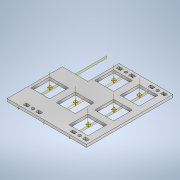
# Autodesk Inventor part: tc_base_plate
Saved by Autodesk Inventor 2020.1 (Build 241239000, 239)
## iProperties
Created: 2019-07-03
Part Number: tc_base_plate
Material: Acier inoxydable
Document SubType Name: Modeling
Designer: Thibault
Density: 8 g/cm^3
Appearance: Aluminium - Poli
Mass: 33.3223 g
Surface Area: 56.2435 cm^2
Volume: 4.16528 cm^3
tc_base_width: 59,100 mm
tc_base_back_width: 40,050 mm
tc_base_support_dist: 56,100 mm
Author: Thibault
Autodesk Inventor part; units mm, degrees
ref_plane "YZ Plane" through (0, 0, 0) normal (1, 0, 0) x (0, 1, 0)
ref_plane "XZ Plane" through (0, 0, 0) normal (0, 1, 0) x (-1, 0, 0)
ref_plane "XY Plane" through (0, 0, 0) normal (0, 0, 1) x (1, 0, 0)
sketch "screw_anchor" plane through (0, 0, 0) normal (0, 0, 1) x (1, 0, 0)
  point P0 (61.1245, 15.5217)
  dimension "d155" = 14
  dimension "d156" = 19.05
  dimension "d157" = 19.05
  dimension "d158" = 19.05
  dimension "d159" = 28.575
  dimension "d160" = 19.05
  dimension "d161" = 2
  dimension "d162" = 2
  dimension "d163" = 2
  dimension "d164" = 2
  dimension "d165" = 2
  dimension "d166" = 1
  dimension "d167" = 5
  dimension "d168" = 5
  dimension "d169" = 4
  dimension "tc_base_support_dist" = 56.1
sketch "anchor" plane through (0, 0, 0) normal (0, 0, 1) x (1, 0, 0)
  circle A0 centre (94.2814, 48.5827) radius 0.85
  line L0 (91.2814, 49.5827) -> (87.2814, 49.5827)
  line L1 (87.2814, 49.5827) -> (87.2814, 47.5827)
  line L2 (87.2814, 47.5827) -> (91.2814, 47.5827)
  line L3 (91.2814, 47.5827) -> (91.2814, 49.5827)
  line L4 (101.2814, 49.5827) -> (97.2814, 49.5827)
  line L5 (97.2814, 49.5827) -> (97.2814, 47.5827)
  line L6 (97.2814, 47.5827) -> (101.2814, 47.5827)
  line L7 (101.2814, 47.5827) -> (101.2814, 49.5827)
  line L8 (91.2814, 49.5827) -> (97.2814, 47.5827) construction
  line L9 (97.2814, 49.5827) -> (91.2814, 47.5827) construction
  line L10 (87.2814, 51.1827) -> (101.2814, 51.1827)
  point P0 (103.5798, 50.1132)
  point P1 (94.2814, 48.5827)
  dimension "tc_base_support_dist" = 56.1
  dimension "d226" = 1.7
  dimension "d230" = 4
  dimension "d231" = 2
  dimension "d237" = 4
  dimension "d245" = 1.6
  dimension "d247" = 6
  measures "d226" diameter of A0
  measures "d230" distance of L2.end L1.end
  measures "d231" distance of L1.end L0.end
  measures "d237" distance of L6.end L5.end
  measures "d245" distance between parallel lines of L0 L10
  measures "d247" distance between parallel lines of L5 L3
sketch "Anchor (screw side)" plane through (0, 0, 0) normal (0, 0, 1) x (1, 0, 0)
  circle A0 centre (93.8994, 50.3042) radius 1.05
  line L0 (90.8494, 51.3542) -> (87.7494, 51.3542)
  line L1 (87.7494, 51.3542) -> (87.7494, 49.2542)
  line L2 (87.7494, 49.2542) -> (90.8494, 49.2542)
  line L3 (90.8494, 49.2542) -> (90.8494, 51.3542)
  line L4 (100.0494, 51.3542) -> (96.9494, 51.3542)
  line L5 (96.9494, 51.3542) -> (96.9494, 49.2542)
  line L6 (96.9494, 49.2542) -> (100.0494, 49.2542)
  line L7 (100.0494, 49.2542) -> (100.0494, 51.3542)
  line L8 (90.8494, 51.3542) -> (96.9494, 49.2542) construction
  line L9 (96.9494, 51.3542) -> (90.8494, 49.2542) construction
  line L10 (85.7494, 53.3542) -> (102.0494, 53.3542) construction
  line L11 (102.0494, 53.3542) -> (102.0494, 47.2542) construction
  line L12 (102.0494, 47.2542) -> (85.7494, 47.2542) construction
  line L13 (85.7494, 47.2542) -> (85.7494, 53.3542) construction
  point P0 (103.5798, 50.1132)
  dimension "d27" = 2.1
  dimension "d28" = 3.1
  dimension "d29" = 2.1
  dimension "slot_distance" = 6.1
  dimension "d34" = 2
  dimension "d35" = 2
  dimension "d36" = 2
  dimension "d37" = 2
  measures "d27" diameter of A0
  measures "d28" distance of L2.end L1.end
  measures "d29" distance of L1.end L0.end
  measures "slot_distance" distance between parallel lines of L5 L3
  measures "d34" distance between parallel lines of L0 L10
  measures "d35" distance between parallel lines of L12 L2
  measures "d36" distance between parallel lines of L11 L7
  measures "d37" distance between parallel lines of L13 L1
sketch "Anchor (nut side)" plane through (0, 0, 0) normal (0, 0, 1) x (1, 0, 0)
  line L0 (11.1, 0) -> (9.1, 0)
  line L1 (9.1, 0) -> (9.1, -2)
  line L2 (9.1, -2) -> (9.9, -2)
  line L3 (9.9, -2) -> (9.9, -4)
  line L4 (6.2, -4) -> (6.2, -2)
  line L5 (6.2, -2) -> (7, -2)
  line L6 (7, -2) -> (7, 0)
  line L7 (7, 0) -> (5, 0)
  line L8 (2, 0) -> (2, 2)
  line L9 (2, 0) -> (3, 0) construction
  line L10 (2, 2) -> (5, 2)
  line L11 (5, 2) -> (5, 0)
  line L12 (11.1, 0) -> (11.1, 2)
  line L13 (11.1, 2) -> (14.1, 2)
  line L14 (14.1, 2) -> (14.1, 0)
  line L15 (0, 0) -> (2, 0)
  line L16 (14.1, 0) -> (16.1, 0)
  line L17 (6.2, -4) -> (7, -4)
  line L18 (9.9, -4) -> (9.1, -4)
  line L19 (7, -4) -> (7, -6.25)
  line L20 (9.1, -4) -> (9.1, -6.25)
  line L21 (7.25, -6.5) -> (8.05, -6.5)
  arc A0 (7, -6.25) -> (7.25, -6.5) centre (7.25, -6.25) ccw
  arc A1 (8.85, -6.5) -> (9.1, -6.25) centre (8.85, -6.25) ccw
  line L22 (8.05, -6.5) -> (8.85, -6.5)
  line L23 (8.05, -3.8983) -> (8.05, -9.959) construction
  point P0 (9.1321, -0.6227)
  point P1 (7, -6.5)
  point P2 (9.1, -6.5)
  dimension "d3" = 2
  dimension "d7" = 6.1
  dimension "d10" = 2
  dimension "d11" = 2
  dimension "d12" = 0.8
  dimension "d13" = 2
  dimension "d14" = 0.8
  dimension "d15" = 2.1
  dimension "d18" = 2
  dimension "d19" = 0.8
  dimension "d20" = 0.8
  dimension "d21" = 2.5
  dimension "d22" = 2.5
  dimension "d23" = 2.1
  dimension "d38" = 2
  dimension "d39" = 0.25
  dimension "d120" = 3
  measures "d3" distance of L15.start L8.start
  measures "d7" distance of L7.end L0.start
  measures "d10" distance of L0.start L0.end
  measures "d11" distance of L0.end L1.end
  measures "d12" distance of L1.end L2.end
  measures "d13" distance of L2.end L3.end
  measures "d14" distance of L4.end L5.end
  measures "d15" distance of L6.end L0.end
  measures "d18" distance of L14.end L16.end
  measures "d19" distance of L4.start L17.end
  measures "d20" distance of L3.end L18.end
  measures "d21" distance of L17.end point (7, -6.5)
  measures "d22" distance of L18.end point (9.1, -6.5)
  measures "d23" distance of L17.end L18.end
  measures "d38" distance between parallel lines of L15 L10
  measures "d39" radius of A0
  measures "d120" distance of L8.end L10.end
sketch "Screwless anchor (male)" plane through (0, 0, 0) normal (0, 0, 1) x (1, 0, 0)
  line L0 (2, 0) -> (2, 2)
  line L1 (2, 0) -> (3, 0) construction
  line L2 (2, 2) -> (5, 2)
  line L3 (5, 2) -> (5, 0)
  line L4 (11.1, 0) -> (11.1, 2)
  line L5 (11.1, 2) -> (14.1, 2)
  line L6 (14.1, 2) -> (14.1, 0)
  line L7 (0, 0) -> (2, 0)
  line L8 (14.1, 0) -> (16.1, 0)
  line L9 (5, 0) -> (11.1, 0)
  point P0 (9.1321, -0.6227)
  dimension "d81" = 2
  dimension "d83" = 6.1
  dimension "d92" = 2
  dimension "d100" = 2
  dimension "d119" = 3
  measures "d81" distance of L7.start L0.start
  measures "d83" distance of L3.end L4.start
  measures "d92" distance of L6.end L8.end
  measures "d100" distance between parallel lines of L7 L2
  measures "d119" distance of L0.end L2.end
sketch "Screwless anchor (female)" plane through (0, 0, 0) normal (0, 0, 1) x (1, 0, 0)
  line L0 (91.7814, 51.7592) -> (88.6814, 51.7592)
  line L1 (88.6814, 51.7592) -> (88.6814, 49.6592)
  line L2 (88.6814, 49.6592) -> (91.7814, 49.6592)
  line L3 (91.7814, 49.6592) -> (91.7814, 51.7592)
  line L4 (100.9814, 51.7592) -> (97.8814, 51.7592)
  line L5 (97.8814, 51.7592) -> (97.8814, 49.6592)
  line L6 (97.8814, 49.6592) -> (100.9814, 49.6592)
  line L7 (100.9814, 49.6592) -> (100.9814, 51.7592)
  line L8 (86.6814, 53.7592) -> (102.9814, 53.7592) construction
  line L9 (102.9814, 53.7592) -> (102.9814, 47.6592) construction
  line L10 (102.9814, 47.6592) -> (86.6814, 47.6592) construction
  line L11 (86.6814, 47.6592) -> (86.6814, 53.7592) construction
  point P0 (103.5798, 50.1132)
  dimension "d106" = 3.1
  dimension "d107" = 2.1
  dimension "d108_1" = 3.1
  dimension "d109_1" = 6.1
  dimension "d110_1" = 2
  dimension "d111_1" = 2
  dimension "d112" = 2
  dimension "d113" = 2
  measures "d106" distance of L2.end L1.end
  measures "d107" distance of L1.end L0.end
  measures "d108_1" distance of L6.end L5.end
  measures "d109_1" distance between parallel lines of L5 L3
  measures "d110_1" distance between parallel lines of L0 L8
  measures "d111_1" distance between parallel lines of L10 L2
  measures "d112" distance between parallel lines of L9 L7
  measures "d113" distance between parallel lines of L11 L1
sketch "Esquisse2" plane through (0, 0, 0) normal (0, 1, 0) x (-1, 0, 0)
  line L0 (17.3848, -3.6295) -> (3.3848, -3.6295)
  line L1 (3.3848, -3.6295) -> (3.3848, 10.3705)
  line L2 (3.3848, 10.3705) -> (17.3848, 10.3705)
  line L3 (17.3848, 10.3705) -> (17.3848, -3.6295)
  line L4 (17.3848, -41.7295) -> (3.3848, -41.7295)
  line L5 (3.3848, -41.7295) -> (3.3848, -27.7295)
  line L6 (3.3848, -27.7295) -> (17.3848, -27.7295)
  line L7 (17.3848, -27.7295) -> (17.3848, -41.7295)
  line L8 (17.3848, -22.6795) -> (3.3848, -22.6795)
  line L9 (3.3848, -22.6795) -> (3.3848, -8.6795)
  line L10 (3.3848, -8.6795) -> (17.3848, -8.6795)
  line L11 (17.3848, -8.6795) -> (17.3848, -22.6795)
  line L12 (36.4348, -41.7295) -> (22.4348, -41.7295)
  line L13 (22.4348, -41.7295) -> (22.4348, -27.7295)
  line L14 (22.4348, -27.7295) -> (36.4348, -27.7295)
  line L15 (36.4348, -27.7295) -> (36.4348, -41.7295)
  line L16 (36.4348, -13.1545) -> (22.4348, -13.1545)
  line L17 (22.4348, -13.1545) -> (22.4348, 0.8455)
  line L18 (22.4348, 0.8455) -> (36.4348, 0.8455)
  line L19 (36.4348, 0.8455) -> (36.4348, -13.1545)
  line L20 (55.4848, -13.1545) -> (41.4848, -13.1545)
  line L21 (41.4848, -13.1545) -> (41.4848, 0.8455)
  line L22 (41.4848, 0.8455) -> (55.4848, 0.8455)
  line L23 (55.4848, 0.8455) -> (55.4848, -13.1545)
  line L24 (57.4848, -24.6795) -> (38.4348, -24.6795)
  line L25 (38.4348, -24.6795) -> (38.4348, -47.8295)
  line L26 (38.4348, -47.8295) -> (-1.6152, -47.8295)
  line L27 (-1.6152, -47.8295) -> (-1.6152, 16.4705)
  line L28 (57.4848, -24.6795) -> (57.4848, 16.4705)
  line L29 (57.4848, 16.4705) -> (-1.6152, 16.4705)
  circle A0 centre (41.3348, 13.4205) radius 1.05
  line L30 (38.2848, 14.4705) -> (35.1848, 14.4705)
  line L31 (35.1848, 14.4705) -> (35.1848, 12.3705)
  line L32 (35.1848, 12.3705) -> (38.2848, 12.3705)
  line L33 (38.2848, 12.3705) -> (38.2848, 14.4705)
  line L34 (47.4848, 14.4705) -> (44.3848, 14.4705)
  line L35 (44.3848, 14.4705) -> (44.3848, 12.3705)
  line L36 (44.3848, 12.3705) -> (47.4848, 12.3705)
  line L37 (47.4848, 12.3705) -> (47.4848, 14.4705)
  line L38 (38.2848, 14.4705) -> (44.3848, 12.3705) construction
  line L39 (44.3848, 14.4705) -> (38.2848, 12.3705) construction
  line L40 (33.1848, 16.4705) -> (49.4848, 16.4705) construction
  line L41 (49.4848, 16.4705) -> (49.4848, 10.3705) construction
  line L42 (49.4848, 10.3705) -> (33.1848, 10.3705) construction
  line L43 (33.1848, 10.3705) -> (33.1848, 16.4705) construction
  circle A1 centre (6.5348, 13.4205) radius 1.05
  line L44 (3.4848, 14.4705) -> (0.3848, 14.4705)
  line L45 (0.3848, 14.4705) -> (0.3848, 12.3705)
  line L46 (0.3848, 12.3705) -> (3.4848, 12.3705)
  line L47 (3.4848, 12.3705) -> (3.4848, 14.4705)
  line L48 (12.6848, 14.4705) -> (9.5848, 14.4705)
  line L49 (9.5848, 14.4705) -> (9.5848, 12.3705)
  line L50 (9.5848, 12.3705) -> (12.6848, 12.3705)
  line L51 (12.6848, 12.3705) -> (12.6848, 14.4705)
  line L52 (3.4848, 14.4705) -> (9.5848, 12.3705) construction
  line L53 (9.5848, 14.4705) -> (3.4848, 12.3705) construction
  line L54 (-1.6152, 16.4705) -> (14.6848, 16.4705) construction
  line L55 (14.6848, 16.4705) -> (14.6848, 10.3705) construction
  line L56 (14.6848, 10.3705) -> (-1.6152, 10.3705) construction
  line L57 (-1.6152, 10.3705) -> (-1.6152, 16.4705) construction
  circle A2 centre (6.5348, -44.7795) radius 1.05
  line L58 (3.4848, -43.7295) -> (0.3848, -43.7295)
  line L59 (0.3848, -43.7295) -> (0.3848, -45.8295)
  line L60 (0.3848, -45.8295) -> (3.4848, -45.8295)
  line L61 (3.4848, -45.8295) -> (3.4848, -43.7295)
  line L62 (12.6848, -43.7295) -> (9.5848, -43.7295)
  line L63 (9.5848, -43.7295) -> (9.5848, -45.8295)
  line L64 (9.5848, -45.8295) -> (12.6848, -45.8295)
  line L65 (12.6848, -45.8295) -> (12.6848, -43.7295)
  line L66 (3.4848, -43.7295) -> (9.5848, -45.8295) construction
  line L67 (9.5848, -43.7295) -> (3.4848, -45.8295) construction
  line L68 (-1.6152, -41.7295) -> (14.6848, -41.7295) construction
  line L69 (14.6848, -41.7295) -> (14.6848, -47.8295) construction
  line L70 (14.6848, -47.8295) -> (-1.6152, -47.8295) construction
  line L71 (-1.6152, -47.8295) -> (-1.6152, -41.7295) construction
  circle A3 centre (30.2848, -44.7795) radius 1.05
  line L72 (27.2348, -43.7295) -> (24.1348, -43.7295)
  line L73 (24.1348, -43.7295) -> (24.1348, -45.8295)
  line L74 (24.1348, -45.8295) -> (27.2348, -45.8295)
  line L75 (27.2348, -45.8295) -> (27.2348, -43.7295)
  line L76 (36.4348, -43.7295) -> (33.3348, -43.7295)
  line L77 (33.3348, -43.7295) -> (33.3348, -45.8295)
  line L78 (33.3348, -45.8295) -> (36.4348, -45.8295)
  line L79 (36.4348, -45.8295) -> (36.4348, -43.7295)
  line L80 (27.2348, -43.7295) -> (33.3348, -45.8295) construction
  line L81 (33.3348, -43.7295) -> (27.2348, -45.8295) construction
  line L82 (22.1348, -41.7295) -> (38.4348, -41.7295) construction
  line L83 (38.4348, -41.7295) -> (38.4348, -47.8295) construction
  line L84 (38.4348, -47.8295) -> (22.1348, -47.8295) construction
  line L85 (22.1348, -47.8295) -> (22.1348, -41.7295) construction
  point P0 (39.3203, -53.3777)
  point P1 (32.3036, -47.8295)
  point P2 (1.2703, -53.3777)
  dimension "tc_base_support_dist" = 56.1
  dimension "d108" = 14
  dimension "d109" = 19.05
  dimension "d110" = 19.05
  dimension "d111" = 19.05
  dimension "d114" = 19.05
  dimension "d123" = 2
  dimension "d181" = 5
  dimension "d190" = 2
  dimension "d258" = 10
  dimension "d260" = 2
  dimension "d263" = 2
  dimension "d269" = 28.575
  dimension "d275" = 2
  constraints: 60 end point, 12 horizontal, 12 parallel, 11 equal length, 7 perpendicular, 6 vertical, 5 collinear, 3 point on line
  measures "d108" distance of L1.end L2.end
  measures "d109" distance of L8.end L4.end
  measures "d110" distance of L0.end L8.end
  measures "d111" distance of L4.start L12.start
  measures "d114" distance of L18.end L22.end
  measures "d123" distance between parallel lines of L8 L24
  measures "d181" distance between parallel lines of L27 L5
  measures "d190" distance between parallel lines of L28 L23
  measures "d269" distance between parallel lines of L16 L12
  measures "d275" distance between parallel lines of L25 L15
extrude "Base" add sketch "Esquisse2" along normal blind 2
ref_plane "Plan de construction4" through (-10.3848, 0, -41.7295) normal (-1, 0, 0) x (0, 0, 1)
ref_plane "Plan de construction5" through (-29.4348, 0, -27.7295) normal (1, 0, 0) x (0, 0, -1)
ref_plane "Plan de construction6" through (-48.4848, 0, -13.1545) normal (-1, 0, 0) x (0, 0, 1)
derived "shared_parameters.ipt"
